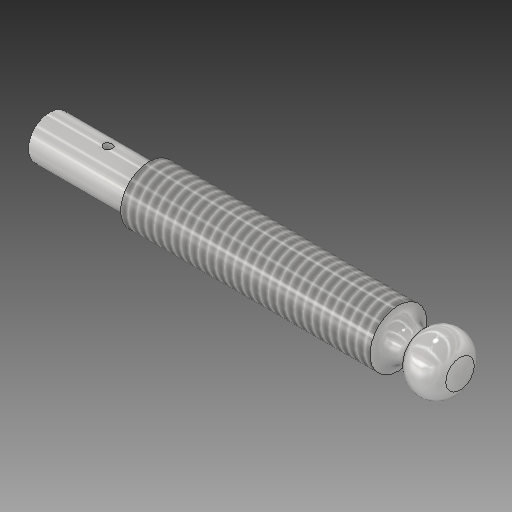
# Autodesk Inventor part: Tornillo de apriete
Saved by Autodesk Inventor 2020 (Build 240168000, 168)
## iProperties
Created: 2016-05-05
Part Number: Tornillo de apriete
Material: Aluminum 6061-AHC
Document SubType Name: Modeling
Designer: Jorge
Mass: 26.2809 g
Surface Area: 35.8189 cm^2
Volume: 9.73367 cm^3
Density: 2.7 g/cm^3
Appearance: Aluminum - Dark
Author: Jorge
Title: Tornillo de apriete
Autodesk Inventor part; units mm, degrees
ref_plane "YZ Plane" through (0, 0, 0) normal (1, 0, 0) x (0, 1, 0)
ref_plane "XZ Plane" through (0, 0, 0) normal (0, 1, 0) x (-1, 0, 0)
sketch "Sketch1" plane through (0, 0, 0) normal (0, 0, 1) x (1, 0, 0)
  line L0 (0, 4.7371) -> (22.225, 4.7371)
  line L1 (22.225, 4.7371) -> (22.225, 6.35)
  line L2 (22.225, 6.35) -> (77.7875, 6.35)
  line L3 (92.075, 6.35) -> (92.075, 0) construction
  line L4 (0, -1.4014) -> (0, 8.4083) construction
  line L5 (-18.7746, 0) -> (112.6474, 0) construction
  line L6 (83.9918, 6.35) -> (93.8728, 6.35) construction
  arc A0 (77.7875, 6.35) -> (83.3836, 4.639) centre (80.946, 6.6733) ccw
  arc A1 (92.075, 0) -> (91.5303, 3.175) centre (82.55, 0) ccw
  arc A2 (91.5303, 3.175) -> (83.3836, 4.639) centre (87.0401, 1.5875) ccw
  line L7 (0, 4.7371) -> (0, 0)
  line L8 (92.075, 0) -> (0, 0)
  dimension "d0" = 92.075
  dimension "d1" = 0
  dimension "d2" = 22.225
  dimension "d3" = 55.5625
  dimension "d4" = 9.4742
  dimension "d5" = 12.7
  dimension "d6" = 12.7
  dimension "d12" = 4.7625
  dimension "d13" = 4.7625
  dimension "d14" = 3.175
  dimension "d15" = 9.525
  constraints: 14 end point, 8 point on circle, 3 centre point, 3 tangent, 2 horizontal, 2 perpendicular, 2 point on line, 1 coincident, 1 collinear, 1 vertical
  measures "d0" distance between parallel lines of L3 L4
  measures "d1" distance from line of L0.start L4
  measures "d2" distance between parallel lines of L1 L4
  measures "d3" distance from line of L2.end L1
  measures "d4" diameter of L0 L5
  measures "d5" diameter of L2 L5
  measures "d6" diameter of L3.start L5
  measures "d12" horizontal distance of A1.centre L2.end
  measures "d13" radius of A2
  measures "d14" radius of A0
  measures "d15" radius of A1
revolve "Revolution1" add sketch "Sketch1" angle 360 about axis through (-10, 0, 0) along (1, 0, 0)
thread "Thread1" size "1/2-13 UNC" class "2A" standard "ANSI Unified Screw Threads" full length
ref_plane "Work Plane1" through (0, 4.7371, 0) normal (0, 1, 0) x (-1, 0, 0)
sketch "Sketch2" plane through (0, 4.7371, 0) normal (0, 1, 0) x (-1, 0, 0)
  point P0 (0, 0)
  point P1 (-13.0485, 0)
hole "Hole1" at (13.0485, 4.7371, 0) direction (0, -1, 0) diameter 1.905 end through all
body "Solid1"
